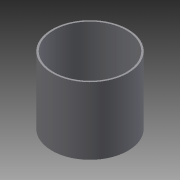
# Autodesk Inventor part: Waveguide Terminator Nipple
Saved by Autodesk Inventor 2014 (Build 180170000, 170)
## iProperties
Created: 2014-05-16
Part Number: Waveguide Terminator Nipple
Material: Generic
Document SubType Name: Modeling
Designer: ijs09
Density: 1 g/cm^3
Appearance: Default
Author: ijs09
Autodesk Inventor part; units mm, degrees
ref_plane "YZ Plane" through (0, 0, 0) normal (1, 0, 0) x (0, 1, 0)
ref_plane "XZ Plane" through (0, 0, 0) normal (0, 1, 0) x (-1, 0, 0)
ref_plane "XY Plane" through (0, 0, 0) normal (0, 0, 1) x (1, 0, 0)
sketch "Sketch1" plane through (0, 0, 0) normal (0, 0, 1) x (1, 0, 0)
  circle A0 centre (0, 0) radius 22.25
  circle A1 centre (0, 0) radius 21.25
  dimension "d0" = 42.5
  dimension "d1" = 44.5
  constraints: 2 centre point, 2 coincident
  measures "d0" diameter of A1
  measures "d1" diameter of A0
extrude "Extrusion1" add sketch "Sketch1" along normal blind 39.4
body "Solid1"
